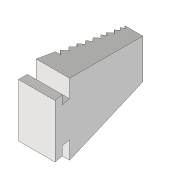
# Autodesk Inventor part: Finger
Saved by Autodesk Inventor 2020 (Build 240168000, 168)
## iProperties
Created: 2020-03-18
Part Number: Finger
Material: Generisch
Document SubType Name: Modeling
Designer: franz
Density: 1 g/cm^3
Appearance: Vorgabe
Author: franz
Autodesk Inventor part; units mm, degrees
ref_plane "YZ Plane" through (0, 0, 0) normal (1, 0, 0) x (0, 1, 0)
ref_plane "XZ Plane" through (0, 0, 0) normal (0, 1, 0) x (-1, 0, 0)
ref_plane "XY Plane" through (0, 0, 0) normal (0, 0, 1) x (1, 0, 0)
sketch "Skizze1" plane through (0, 0, 0) normal (1, 0, 0) x (0, 1, 0)
  line L0 (-10, -10) -> (-10, -5)
  line L1 (-10, -5) -> (-15, -5)
  line L2 (-15, -5) -> (-15, 0)
  line L3 (-15, 0) -> (15, 0)
  line L4 (15, 0) -> (15, -5)
  line L5 (15, -5) -> (10, -5)
  line L6 (10, -5) -> (10, -10)
  line L7 (10, -10) -> (20, -10)
  line L8 (20, -10) -> (11.1837, -60)
  line L9 (11.1837, -60) -> (-11.1837, -60)
  line L10 (-11.1837, -60) -> (-20, -10)
  line L11 (-20, -10) -> (-10, -10)
  line L12 (0, -72) -> (0, 12) projected
  point P0 (0, 0)
  dimension "d0" = 30
  dimension "d1" = 20
  dimension "d2" = 5
  dimension "d3" = 5
  dimension "d4" = 50
  dimension "d5" = 80
  dimension "d6" = 40
  constraints: 24 end point, 5 perpendicular, 2 parallel, 1 collinear, 1 midpoint, 1 point on line, 1 vertical, 5 other
  measures "d0" distance of L2.end L3.end
  measures "d1" distance between parallel lines of L6 L0
  measures "d2" distance of L1.end L2.end
  measures "d3" distance of L0.start L0.end
  measures "d4" distance between parallel lines of L11 L9
  measures "d5" angle of L7 L8
  measures "d6" distance of L7.end L10.end
extrude "Extrusion1" add sketch "Skizze1" along normal blind 10
draft "Flächenverjüngung1" angle 10 pull direction (0, 0, -1) faces at (10, -3.3333, -43.3333) fixed edges at (10, 0, -60)
sketch "Skizze2" plane through (0, -15, -5) normal (0, -1, 0) x (1, 0, 0)
  line L0 (0, -55) -> (10, -55) projected
  line L1 (0, -55) -> (0, -15.878)
  line L2 (0, -5) -> (0, -55) projected
  line L3 (0, -15.878) -> (2.7928, -15.878)
  line L4 (2.7928, -15.878) -> (0, -18.411)
  line L5 (2.4331, -21.0937) -> (0, -23.3005)
  line L6 (1.8286, -26.2976) -> (0, -27.9561)
  line L7 (0, -18.411) -> (2.4331, -21.0937)
  line L8 (0, -23.3005) -> (1.8286, -26.2976)
  line L9 (0, -27.9561) -> (2.0847, -30.4266)
  line L10 (2.0847, -30.4266) -> (0, -32.9397)
  line L11 (0, -55) -> (0, -5) projected
  line L12 (0, -32.9397) -> (2.1741, -34.4602)
  line L13 (2.1741, -34.4602) -> (0, -37.1114)
  line L14 (0, -37.1114) -> (1.9385, -39.4086)
  line L15 (1.9385, -39.4086) -> (0, -41.407)
  line L16 (0, -41.407) -> (1.9544, -43.0098)
  line L17 (1.9544, -43.0098) -> (0, -44.659)
  line L18 (0, -44.659) -> (2.0679, -47.1635)
  line L19 (2.0679, -47.1635) -> (0, -48.8464)
  line L20 (0, -48.8464) -> (1.614, -50.6034)
  line L21 (1.614, -50.6034) -> (0, -52.2673)
  line L22 (0, -52.2673) -> (1.8319, -53.7695)
  line L23 (1.8319, -53.7695) -> (0, -55)
  point P0 (0, 5)
  point P1 (0, -52.2673)
  point P2 (0, -52.2673)
  constraints: 42 end point, 10 point on line, 5 parallel, 2 perpendicular, 1 horizontal, 3 other
extrude "Extrusion2" cut sketch "Skizze2" along normal through all both and the other way through all
